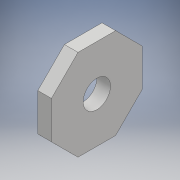
# Autodesk Inventor part: Nuy
Saved by Autodesk Inventor 2018 (Build 220112000, 112)
## iProperties
Created: 2019-05-13
Part Number: Nuy
Material: Generic
Document SubType Name: Modeling
Designer: aal_9
Density: 1 g/cm^3
Appearance: Default
Author: aal_9
Autodesk Inventor part; units mm, degrees
ref_plane "YZ Plane" through (0, 0, 0) normal (1, 0, 0) x (0, 1, 0)
ref_plane "XZ Plane" through (0, 0, 0) normal (0, 1, 0) x (-1, 0, 0)
ref_plane "XY Plane" through (0, 0, 0) normal (0, 0, 1) x (1, 0, 0)
sketch "Sketch1" plane through (0, 0, 0) normal (1, 0, 0) x (0, 1, 0)
  line L0 (-4.1396, 10.001) -> (4.1446, 9.999)
  line L1 (4.1446, 9.999) -> (10.001, 4.1396)
  line L2 (10.001, 4.1396) -> (9.999, -4.1446)
  line L3 (9.999, -4.1446) -> (4.1396, -10.001)
  line L4 (4.1396, -10.001) -> (-4.1446, -9.999)
  line L5 (-4.1446, -9.999) -> (-10.001, -4.1396)
  line L6 (-10.001, -4.1396) -> (-9.999, 4.1446)
  line L7 (-9.999, 4.1446) -> (-4.1396, 10.001)
  circle A0 centre (0, 0) radius 3
  dimension "d0" = 10
  dimension "d1" = 6
  constraints: 16 end point, 2 coincident, 1 centre point, 17 other
  measures "d0" distance from line of L2 point (0, 0)
  measures "d1" diameter of A0
extrude "Extrusion1" add sketch "Sketch1" along normal blind 3
body "Solid1"
